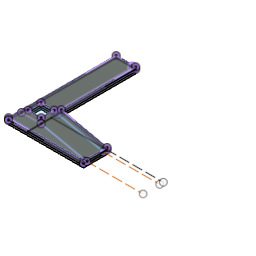
coin-guide_3D (Autodesk Fusion 360 design; units mm, degrees)
Autodesk Fusion 360 part; units mm, degrees
note: some values were not read from the file. Set by a fixed rule: which sketch regions a step uses.
sketch "Sketch1" plane through (0, 0, 0) normal (0, 0, 1) x (1, 0, 0)
  line L0 (0, 0) -> (30, 0)
  line L1 (30, 0) -> (30, 165)
  line L2 (30, 165) -> (0, 165)
  line L3 (0, 165) -> (0, 0)
  line L4 (30, 0) -> (115, 0)
  line L5 (115, 0) -> (115, 36)
  line L6 (115, 36) -> (30, 36)
  line L7 (30, 36) -> (30, 0)
  line L8 (115, 5) -> (30, 19.9878)
  line L9 (115, 5) -> (201.3113, 5) construction
  line L10 (115, 30.5) -> (30, 45.4878)
  line L11 (115, 30.5) -> (201.3113, 30.5) construction
  line L12 (115, 36) -> (30, 50.9878)
  line L13 (115, 36) -> (201.3113, 36) construction
  dimension "d1" = 30
  dimension "d2" = 165
  dimension "d3" = 85
  dimension "d4" = 36
  dimension "d5" = 170
  dimension "d6" = 170
  dimension "d7" = 170
  constraint horizontal L0
  constraint vertical L1
  constraint horizontal L2
  constraint vertical L3
  constraint coincident L0.start L3.end
  constraint horizontal L4
  constraint vertical L5
  constraint horizontal L6
  constraint vertical L7
  constraint horizontal L9
  constraint coincident L5 L8.start
  constraint coincident L7 L8.end
  constraint horizontal L11
  constraint coincident L5 L10.start
  constraint coincident L1 L10.end
  constraint horizontal L13
  constraint coincident L1 L12.end
  measures "d1" distance of L0.start L0.end
  measures "d2" distance of L0.start L2.end
  measures "d3" distance of L0.end L4.end
  measures "d4" distance of L0.end L6.end
  measures "d5" angle of L8 L9
  measures "d6" angle of L10 L11
  measures "d7" angle of L12 L13
extrude "Extrude1" add sketch "Sketch1" along normal blind 3 makes body 1
sketch "Sketch3" plane through (0, 0, 3) normal (0, 0, 1) x (-1, 0, 0)
  line L0 (-115, -36) -> (-30, -50.9878)
  line L1 (-30, -50.9878) -> (-30, -165)
  line L2 (-30, -165) -> (0, -165)
  line L3 (0, -165) -> (0, 0)
  line L4 (0, 0) -> (-115, 0)
  line L5 (-115, 0) -> (-115, -36)
  line L6 (-5, -25) -> (-25, -25)
  line L7 (-25, -25) -> (-25, -45)
  line L8 (-25, -45) -> (-5, -45)
  line L9 (-5, -45) -> (-5, -25)
  dimension "d10" = 20
  dimension "d11" = 20
  constraint horizontal L6
  constraint vertical L7
  constraint horizontal L8
  constraint vertical L9
  measures "d10" distance of L6.start L6.end
  measures "d11" distance of L6.start L8.end
extrude "Extrude2" cut sketch "Sketch3" against normal blind 3 contours L6 L7 L8 L9 bodies 1
sketch "coin guide 1" plane through (0, 0, 3) normal (0, 0, 1) x (-1, 0, 0)
  line L0 (-25, -25) -> (-5, -25)
  line L1 (-5, -25) -> (-5, -45)
  line L2 (-5, -45) -> (-25, -45)
  line L3 (-25, -45) -> (-25, -25)
  line L4 (-115, -36) -> (-30, -50.9878)
  line L5 (-30, -50.9878) -> (-30, -165)
  line L6 (-30, -165) -> (0, -165)
  line L7 (0, -165) -> (0, 0)
  line L8 (0, 0) -> (-115, 0)
  line L9 (-115, 0) -> (-115, -36)
sketch "Sketch5" plane through (0, 0, 0) normal (0, 0, 1) x (1, 0, 0)
  line L0 (0, 0) -> (30, 0)
  line L1 (30, 0) -> (30, 20)
  line L2 (30, 20) -> (0, 20)
  line L3 (0, 20) -> (0, 0)
  line L4 (30, 45.4878) -> (25, 45.4878)
  line L5 (25, 45.4878) -> (25, 165)
  line L6 (25, 165) -> (30, 165)
  line L7 (30, 165) -> (30, 45.4878)
  line L8 (30, 165) -> (0, 165)
  line L9 (25, 165) -> (0, 165)
  line L10 (0, 165) -> (0, 160)
  line L11 (25, 160) -> (25, 165)
  point P0 (30, 45.4878)
  dimension "d14" = 5
  dimension "d17" = 25
  dimension "d18" = 5
  constraint horizontal L0
  constraint vertical L1
  constraint horizontal L2
  constraint vertical L3
  constraint coincident L0.start L3.end
  constraint horizontal L4
  constraint vertical L5
  constraint horizontal L6
  constraint vertical L7
  constraint coincident L5.end L8
  constraint coincident P0 L4.start
  constraint horizontal L9
  constraint vertical L10
  constraint vertical L11
  measures "d14" distance of P0 L4.end
  measures "d17" distance of L5.end L8.end
  measures "d18" distance of L5.end L11.start
extrude "Extrude3" add sketch "Sketch5" sketch "Sketch1" against normal blind 3 separate body of sketch 2 contours L1 L4 L5 L7 L8 | L1 L6 L10 L12 | L5 L6 L10 makes body 2 at (58.3333, 44.1585, 0) makes body 3 at (48.3333, 6.6626, 0)
copy_body "CopyPasteBodies1" bodies 1 makes body 4
move_body "Move1" bodies 4 to x (1, 0, 0) y (0, 1, 0) z (0, 0, 1) at (0, 0, -6)
sketch "coin guide 2.1" plane through (0, 0, 0) normal (0, 0, 1) x (-1, 0, 0)
  line L0 (-30, -165) -> (-25, -165)
  line L1 (-25, -165) -> (-25, -45.4878)
  line L2 (-25, -45.4878) -> (-30, -45.4878)
  line L3 (-30, -45.4878) -> (-115, -30.5)
  line L4 (-115, -30.5) -> (-115, -36)
  line L5 (-115, -36) -> (-30, -50.9878)
  line L6 (-30, -50.9878) -> (-30, -165)
sketch "coin guide 2.2" plane through (0, 0, 0) normal (0, 0, 1) x (-1, 0, 0)
  line L0 (0, -20) -> (0, 0)
  line L1 (0, 0) -> (-115, 0)
  line L2 (-115, 0) -> (-115, -5)
  line L3 (-115, -5) -> (-30, -19.9878)
  line L4 (-30, -19.9878) -> (-30, -20)
  line L5 (-30, -20) -> (0, -20)
